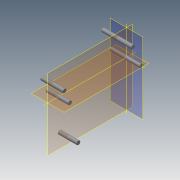
# Autodesk Inventor part: HbIndexPosture_flex01
Saved by Autodesk Inventor 2015 SP1 (Build 190203100, 203)
## iProperties
Created: 2015-02-13
Part Number: HbIndexPosture_flex01
Material: 一般
Document SubType Name: Modeling
Designer: Yamaura
Density: 1 g/cm^3
Appearance: 既定
Author: Yamaura
Autodesk Inventor part; units mm, degrees
sketch "スケッチ1" plane through (0, 0, 0) normal (1, 0, 0) x (0, 1, 0)
  circle A0 centre (0, 0) radius 1
  circle A1 centre (-36.4, 0) radius 1
  circle A2 centre (-30.8913, -21.8152) radius 1
  line L0 (-36.4, 0) -> (0, 0)
  line L1 (-30.8913, -21.8152) -> (-36.4, 0)
  line L2 (0, 0) -> (0, 70.9009)
  circle A3 centre (-4.5922, 11.0866) radius 1
  circle A4 centre (-39.3028, 7.0024) radius 1
  line L3 (0, 0) -> (-4.5922, 11.0866)
  line L4 (-39.3028, 7.0024) -> (-36.4, 0)
  line L5 (-39.3028, 7.0024) -> (-4.5922, 11.0866)
  line L6 (-48.5633, 0) -> (9.2606, 0) projected
  line L7 (-39.3028, 7.0024) -> (-38.2362, 7.2717)
  line L8 (-36.4, 0) -> (-38.2362, 7.2717)
  line L9 (0, 0) -> (0, 28.7676)
  dimension "d0" = 2
  dimension "d1" = 2
  dimension "d2" = 2
  dimension "d3" = 36.4
  dimension "d4" = 22.5
  dimension "d5" = 90
  dimension "d9" = 2
  dimension "d10" = 2
  dimension "d13" = 12
  dimension "d15" = 34.95
  dimension "d23" = 1.1
  dimension "d24" = 7.5
  dimension "d29" = 90
  dimension "d30" = 22.5
  constraints: 18 end point, 5 centre point, 2 coincident, 2 vertical, 1 collinear, 1 perpendicular
  measures "d0" diameter of A0
  measures "d1" diameter of A1
  measures "d2" diameter of A2
  measures "d3" distance of L0.start L0.end
  measures "d4" distance of L1.start L0.start
  measures "d5" angle of L0 L2
  measures "d9" diameter of A3
  measures "d10" diameter of A4
  measures "d13" distance of L0.end L3.end
  measures "d15" distance of L4.start L3.end
  measures "d23" distance from line of L1 A4.centre
  measures "d24" distance of L0.start L7.end
  measures "d29" angle of L0 L9
  measures "d30" angle of L9 L3
extrude "押し出し1" add sketch "スケッチ1" along normal mid plane 10 contours L6 L2 A0 | A0 L0 L6 | L2 L3 A0 | A0 L3 L0 | L0 L8 A1 | A1 L1 L0 | L3 L5 A3 | A3 L5 L3 | L8 L4 A1 | A1 L6 L1 | L6 A1 L4 | L4 L5 A4 | A4 L7 L4 | L5 L7 A4 | A2
move faces "移動1" translate (3, 0, 0) faces at (5, -5.0742, 10.9876) (5, 0.5848, -0.397) (3.3333, 0.9871, -0.1604) (-3.3333, 0.9871, -0.1604)
move faces "移動2" translate (-3, 0, 0) faces at (-5, -5.0742, 10.9876) (-5, 0.5848, -0.397)
move faces "移動3" translate (1, 0, 0) faces at (5, -39.7818, 6.7248) (5, -36.7299, -0.221)
move faces "移動4" translate (-1, 0, 0) faces at (-5, -39.7818, 6.7248) (-5, -36.7299, -0.221)
